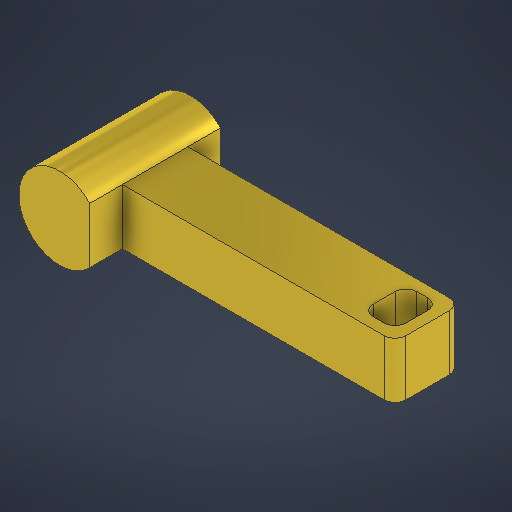
# Autodesk Inventor part: Part2final
Saved by Autodesk Inventor 2026 (Build 300175050, 175E)
## iProperties
Created: 2026-05-04
Part Number: Part2final
Material: Generic
Document SubType Name: Modeling
Designer: ptp527
Density: 1 g/cm^3
Appearance: Default
Author: ptp527
Autodesk Inventor part; units mm, degrees
ref_plane "YZ Plane" through (0, 0, 0) normal (1, 0, 0) x (0, 1, 0)
ref_plane "XZ Plane" through (0, 0, 0) normal (0, 1, 0) x (-1, 0, 0)
ref_plane "XY Plane" through (0, 0, 0) normal (0, 0, 1) x (1, 0, 0)
sketch "Sketch1" plane through (0, 0, 0) normal (0, 0, 1) x (1, 0, 0)
  circle A0 centre (0, 0) radius 75
  dimension "d0" = 150
  constraints: 1 centre point, 1 coincident
  measures "d0" diameter of A0
extrude "Extrusion1" add sketch "Sketch1" along normal blind 240
sketch "Sketch2" plane through (0, 0, 240) normal (0, 0, 1) x (1, 0, 0)
  line L0 (95, -87.5905) -> (55, -87.5905)
  line L1 (55, -87.5905) -> (55, 87.5905)
  line L2 (55, 87.5905) -> (95, 87.5905)
  line L3 (95, 87.5905) -> (95, -87.5905)
  circle A0 centre (0, 0) radius 75 projected
  line L4 (95, -87.5905) -> (55, 87.5905) construction
  line L5 (55, -87.5905) -> (95, 87.5905) construction
  point P0 (75, 0)
  point P1 (55, 50.9902)
  point P2 (55, -50.9902)
  dimension "d3" = 40
  constraints: 12 end point, 2 midpoint, 2 parallel, 1 horizontal, 1 perpendicular, 2 other
  measures "d3" distance of L1.end L2.end
extrude "Extrusion2" cut sketch "Sketch2" against normal blind 240 contours L1 A0 picked at (65.2118, -7.3649)
sketch "Sketch3" plane through (55, -50.9902, 240) normal (1, 0, 0) x (0, 0, -1)
  line L0 (0, 101.9804) -> (240, 101.9804) projected
  line L1 (59.9997, -0.0764) -> (179.9997, -0.0764)
  line L2 (179.9997, -0.0764) -> (179.9997, 101.9804)
  line L3 (179.9997, 101.9804) -> (59.9997, 101.9804)
  line L4 (59.9997, 101.9804) -> (59.9997, -0.0764)
  line L5 (59.9997, -0.0764) -> (179.9997, 101.9804) construction
  line L6 (179.9997, -0.0764) -> (59.9997, 101.9804) construction
  point P0 (240, 50.9902)
  point P1 (119.9997, 50.952)
  point P2 (59.9997, 101.9804)
  dimension "d6" = 240
  dimension "d7" = 60
  dimension "d8" = 102.0568
  constraints: 12 end point, 2 midpoint, 2 parallel, 1 horizontal, 1 perpendicular, 1 point on line
  measures "d6" distance of L0.start L0.end
  measures "d7" distance from line of L4 point (120, 50.952)
  measures "d8" distance of L3.end L1.start
extrude "Extrusion3" add sketch "Sketch3" along normal blind 500
sketch "Sketch4" plane through (55, 50.9902, 180.0003) normal (0, 1, 0) x (1, 0, 0)
  line L0 (420, 20) -> (480, 20)
  line L1 (480, 20) -> (480, 100)
  line L2 (480, 100) -> (420, 100)
  line L3 (420, 100) -> (420, 20)
  line L4 (420, 20) -> (480, 100) construction
  line L5 (480, 20) -> (420, 100) construction
  line L6 (0, 120) -> (500, 120) projected
  line L7 (500, 120) -> (500, 0) projected
  point P0 (-55, 180.0003)
  point P1 (450, 60)
  dimension "d11" = 80
  dimension "d12" = 40
  dimension "d13" = 60
  dimension "d14" = 20
  dimension "d15" = 60
  constraints: 12 end point, 2 midpoint, 2 parallel, 1 horizontal, 1 perpendicular
  measures "d11" distance of L0.end L1.end
  measures "d12" distance from line of point (450, 60) L2
  measures "d13" distance from line of L6 point (450, 60)
  measures "d14" distance between parallel lines of L7 L1
  measures "d15" distance between parallel lines of L1 L3
extrude "Extrusion4" cut sketch "Sketch4" along normal mid plane 500
fillet "Fillet1" radius 20 2 edges at (555, -0.0382, 60.0003) (555, -0.0382, 180.0003)
fillet "Fillet2" radius 20 4 edges at (535, -0.0382, 160.0003) (535, -0.0382, 80.0003) (475, -0.0382, 160.0003) (475, -0.0382, 80.0003)
body "Solid1"
